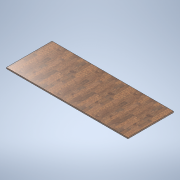
# Autodesk Inventor part: Table
Saved by Autodesk Inventor 2020 (Build 240168000, 168)
## iProperties
Created: 2019-11-09
Part Number: Table
Material: Generic
Document SubType Name: Modeling
Designer: nicoc
Density: 1 g/cm^3
Appearance: White Ash - Java
Author: nicoc
Autodesk Inventor part; units mm, degrees
ref_plane "YZ Plane" through (0, 0, 0) normal (1, 0, 0) x (0, 1, 0)
ref_plane "XZ Plane" through (0, 0, 0) normal (0, 1, 0) x (-1, 0, 0)
ref_plane "XY Plane" through (0, 0, 0) normal (0, 0, 1) x (1, 0, 0)
sketch "Sketch1" plane through (0, 0, 0) normal (0, 1, 0) x (-1, 0, 0)
  line L0 (0, 0) -> (2000, 0)
  line L1 (2000, 0) -> (2000, -750)
  line L2 (2000, -750) -> (0, -750)
  line L3 (0, -750) -> (0, 0)
  dimension "d0" = 750
  dimension "d1" = 2000
  constraints: 8 end point, 2 parallel, 1 horizontal, 1 perpendicular
  measures "d0" distance between parallel lines of L2 L0
  measures "d1" distance between parallel lines of L1 L3
extrude "Extrusion1" add sketch "Sketch1" along normal blind 20
body "Solid1"
